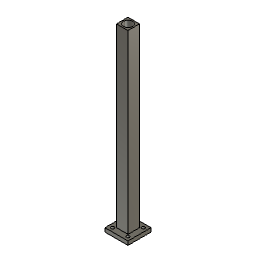
Sensor_mount (Autodesk Fusion 360 design; units mm, degrees)
part number: 2025-07-07-11-45-10-913
part number: 2025-07-07-11-53-10-641
Autodesk Fusion 360 part; units mm, degrees
sketch "Sketch1" plane through (0, 0, 0) normal (0, 0, 1) x (1, 0, 0) in component "Holder"
  line L0 (0, 0) -> (30, 0)
  line L1 (30, 0) -> (30, 30)
  line L2 (30, 30) -> (0, 30)
  line L3 (0, 30) -> (0, 0)
  circle A0 centre (5, 25) radius 2
  circle A1 centre (5, 5) radius 2
  circle A2 centre (25, 25) radius 2
  circle A3 centre (25, 5) radius 2
  dimension "d1" = 30
  dimension "d2" = 30
  dimension "d4" = 4
  dimension "d5" = 4
  dimension "d6" = 20
  dimension "d7" = 5
  dimension "d8" = 5
  dimension "d9" = 4
  dimension "d10" = 20
  dimension "d11" = 5
  dimension "d12" = 4
  dimension "d13" = 20
  dimension "d14" = 20
  constraint horizontal L0
  constraint vertical L1
  constraint horizontal L2
  constraint vertical L3
  constraint coincident L0.start L3.end
  measures "d1" distance of L0.start L0.end
  measures "d2" distance of L0.start L2.end
  measures "d4" diameter of A0
  measures "d5" diameter of A1
  measures "d6" distance of A0.centre A1.centre
  measures "d7" distance of L2 A0.centre
  measures "d8" distance of L0 A1.centre
  measures "d9" diameter of A2
  measures "d10" distance of A0.centre A2.centre
  measures "d11" distance of L2 A2.centre
  measures "d12" diameter of A3
  measures "d13" distance of A1.centre A3.centre
  measures "d14" distance of A2.centre A3.centre
extrude "Extrude1" add sketch "Sketch1" along normal blind 5 in component "Holder"
sketch "Sketch2" plane through (0, 0, 5) normal (0, 0, 1) x (-1, 0, 0) in component "Holder"
  circle A0 centre (-5, -5) radius 2
  circle A1 centre (-25, -5) radius 2
  circle A2 centre (-5, -25) radius 2
  circle A3 centre (-25, -25) radius 2
  line L0 (0, -30) -> (0, 0)
  line L1 (0, 0) -> (-30, 0)
  line L2 (-30, 0) -> (-30, -30)
  line L3 (-30, -30) -> (0, -30)
  line L4 (-7.5, -22.5) -> (-22.5, -22.5)
  line L5 (-22.5, -22.5) -> (-22.5, -7.5)
  line L6 (-22.5, -7.5) -> (-7.5, -7.5)
  line L7 (-7.5, -7.5) -> (-7.5, -22.5)
  circle A4 centre (-15, -15) radius 5.9
  dimension "d17" = 15
  dimension "d18" = 15
  dimension "d19" = 7.5
  dimension "d20" = 7.5
  dimension "d21" = 11.8
  dimension "d22" = 15
  constraint horizontal L4
  constraint vertical L5
  constraint horizontal L6
  constraint vertical L7
  measures "d17" distance of L4.start L4.end
  measures "d18" distance of L4.start L6.end
  measures "d19" distance of L3 L4
  measures "d20" distance of L0 L7
  measures "d21" diameter of A4
  measures "d22" distance of L2 A4.centre
extrude "Extrude2" add sketch "Sketch2" along normal blind 30 contours L4 L5 L6 L7 in component "Holder"
extrude "Extrude3" add 1 faces at (15.147, 8.0388, 35) along direction (0, 0, 1) blind 2 in component "Holder"
extrude "Extrude4" add 1 faces at (15.147, 8.0388, 37) along direction (0, 0, 1) blind 18 in component "Holder"
extrude "Extrude5" add 1 faces at (15.147, 8.0388, 55) along direction (0, 0, 1) blind 180 in component "Holder"
component "Holder" placed x (1, 0, 0) y (0, 1, 0) z (0, 0, 1) at (0, 0, 0)
